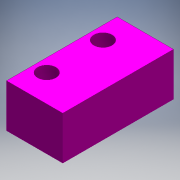
# Autodesk Inventor part: Endstop_Fixture
Saved by Autodesk Inventor 2016 (Build 200138000, 138)
## iProperties
Created: 2015-08-05
Part Number: Endstop_Fixture
Material: Generic
Document SubType Name: Modeling
Designer: 3DPrinterUser
Density: 1 g/cm^3
Appearance: Magenta
Author: 3DPrinterUser
Autodesk Inventor part; units mm, degrees
ref_plane "YZ Plane" through (0, 0, 0) normal (1, 0, 0) x (0, 1, 0)
ref_plane "XZ Plane" through (0, 0, 0) normal (0, 1, 0) x (-1, 0, 0)
ref_plane "XY Plane" through (0, 0, 0) normal (0, 0, 1) x (1, 0, 0)
derived "Endstop.ipt"
sketch "Sketch1" plane through (0, 0, 0) normal (0, 0, 1) x (1, 0, 0)
  line L0 (-3.25, 6.4) -> (3.25, 6.4)
  line L1 (3.25, 6.4) -> (3.25, -6.4)
  line L2 (3.25, -6.4) -> (-3.25, -6.4)
  line L3 (-3.25, -6.4) -> (-3.25, 6.4)
  line L4 (-3.25, 6.4) -> (3.25, -6.4) construction
  line L5 (3.25, 6.4) -> (-3.25, -6.4) construction
  line L6 (3.25, -6.4) -> (3.25, 6.4)
  line L7 (3.25, 6.4) -> (6.25, 6.4)
  line L8 (6.25, 6.4) -> (6.25, -11.6)
  line L9 (6.25, -11.6) -> (3.25, -11.6)
  line L10 (3.25, -11.6) -> (3.25, 6.4)
  line L11 (-3.25, 6.4) -> (-6.55, 6.4)
  line L12 (-6.55, 6.4) -> (-6.55, -6.4)
  line L13 (-6.55, -6.4) -> (-3.25, -6.4)
  line L14 (-3.25, -6.4) -> (-3.25, 6.4)
  line L15 (3.25, 0) -> (-3.25, 0) construction
  point P0 (0, 0)
  point P1 (-1.75, -3.25)
  point P2 (-1.75, 3.25)
extrude "Extrusion1" add sketch "Sketch1" along normal blind 5 contours L0 L1 L2 L3
hole "Hole1" at (-1.75, -3.25, 0) at (-1.75, 3.25, 0) direction (0, 0, 1) diameter 2.1 end through all
body "Solid1"
